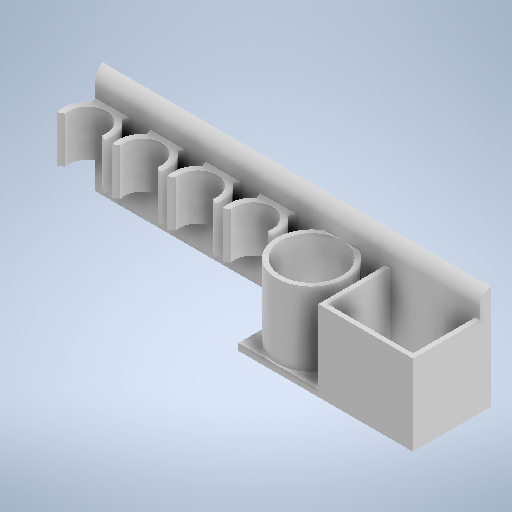
# Autodesk Inventor part: Block-1
Saved by Autodesk Inventor 2025 (Build 290162000, 162)
## iProperties
Created: 2024-07-25
Part Number: Block-1
Material: Generic
Document SubType Name: Modeling
Designer: ethan
Density: 1 g/cm^3
Appearance: Default
Author: ethan
Autodesk Inventor part; units mm, degrees
ref_plane "YZ Plane" through (0, 0, 0) normal (1, 0, 0) x (0, 1, 0)
ref_plane "XZ Plane" through (0, 0, 0) normal (0, 1, 0) x (-1, 0, 0)
ref_plane "XY Plane" through (0, 0, 0) normal (0, 0, 1) x (1, 0, 0)
sketch "Sketch1" plane through (0, 0, 0) normal (0, 1, 0) x (-1, 0, 0)
  arc A0 (-1.6722, -8.0788) -> (-1.6722, 8.0788) centre (0, 0) ccw
  arc A1 (-2.9725, -10.3309) -> (-2.9725, 10.3309) centre (0, 0) ccw
  line L0 (-1.6722, 8.0788) -> (-2.9725, 10.3309)
  line L1 (-1.6722, 8.0788) -> (0.9283, 8.0788) construction
  line L2 (-1.6722, -8.0788) -> (-2.9725, -10.3309)
  line L3 (0, 0) -> (0, -2.9706)
  arc A2 (-1.6722, -32.0788) -> (-1.6722, -15.9212) centre (0, -24) ccw
  arc A3 (-2.9725, -34.3309) -> (-2.9725, -13.6691) centre (0, -24) ccw
  line L4 (-1.6722, -15.9212) -> (-2.9725, -13.6691)
  line L5 (-1.6722, -15.9212) -> (0.9283, -15.9212) construction
  line L6 (-1.6722, -32.0788) -> (-2.9725, -34.3309)
  line L7 (0, -24) -> (0, -26.9706)
  arc A4 (-1.6722, -56.0788) -> (-1.6722, -39.9212) centre (0, -48) ccw
  arc A5 (-2.9725, -58.3309) -> (-2.9725, -37.6691) centre (0, -48) ccw
  line L8 (-1.6722, -39.9212) -> (-2.9725, -37.6691)
  line L9 (-1.6722, -39.9212) -> (0.9283, -39.9212) construction
  line L10 (-1.6722, -56.0788) -> (-2.9725, -58.3309)
  line L11 (0, -48) -> (0, -50.9706)
  arc A6 (-1.6722, -80.0788) -> (-1.6722, -63.9212) centre (0, -72) ccw
  arc A7 (-2.9725, -82.3309) -> (-2.9725, -61.6691) centre (0, -72) ccw
  line L12 (-1.6722, -63.9212) -> (-2.9725, -61.6691)
  line L13 (-1.6722, -63.9212) -> (0.9283, -63.9212) construction
  line L14 (-1.6722, -80.0788) -> (-2.9725, -82.3309)
  line L15 (0, -72) -> (0, -74.9706)
  line L16 (10.75, -99.7274) -> (-2.45, -99.7274) construction
  circle A8 centre (-2.45, -99.7274) radius 13.2 construction
  arc A9 (10.75, -92.1908) -> (10.75, -107.264) centre (-2.45, -99.7274) ccw construction
  circle A10 centre (-2.45, -99.7274) radius 13.2
  arc A11 (10.75, -92.1908) -> (10.75, -107.264) centre (-2.45, -99.7274) ccw
  line L17 (10.75, -120.472) -> (-16.25, -120.472)
  line L18 (-16.25, -120.472) -> (-16.25, -157.572)
  line L19 (-16.25, -157.572) -> (10.75, -157.572)
  line L20 (10.75, -157.572) -> (10.75, -120.472)
  line L21 (-18.25, -159.572) -> (-18.25, -118.472)
  line L22 (-18.25, -118.472) -> (10.75, -118.472)
  line L23 (12.75, -159.572) -> (-18.25, -159.572)
  line L24 (10.75, 0) -> (15.75, 0) construction
  line L25 (8.4709, 6.6186) -> (15.75, 9.268) construction
  line L26 (15.75, 9.268) -> (15.75, -159.572) construction
  line L27 (15.75, -159.572) -> (12.75, -159.572) construction
  line L28 (10.75, -118.472) -> (10.75, -107.264) construction
  line L29 (10.75, -118.472) -> (10.75, -107.264)
  line L30 (10.75, -92.1908) -> (10.75, -79.8019)
  line L31 (8.4709, 6.6186) -> (15.75, 9.268)
  line L32 (15.75, 9.268) -> (15.75, -159.572)
  line L33 (15.75, -159.572) -> (12.75, -159.572)
  line L34 (10.75, -107.264) -> (10.75, -118.472) construction
  line L35 (10.75, -120.472) -> (10.75, -154.7804) construction
  line L36 (8.4709, -6.6186) -> (10.75, -7.4481)
  line L37 (8.4709, -6.6186) -> (10.8963, -6.6186) construction
  line L38 (8.4709, -17.3814) -> (10.75, -16.5519)
  line L39 (8.4709, -30.6186) -> (10.75, -31.4481)
  line L40 (8.4709, -41.3814) -> (10.75, -40.5519)
  line L41 (8.4709, -54.6186) -> (10.75, -55.4481)
  line L42 (8.25, -65.108) -> (10.75, -64.1981)
  line L43 (8.25, -78.892) -> (10.75, -79.8019)
  line L44 (10.75, -16.5519) -> (10.75, -7.4481)
  line L45 (10.75, -7.4481) -> (10.75, -16.5519) construction
  line L46 (10.75, -64.1981) -> (10.75, -55.4481)
  line L47 (10.75, -40.5519) -> (10.75, -31.4481)
  line L48 (10.75, -31.4481) -> (10.75, -40.5519) construction
  line L49 (10.75, -55.4481) -> (10.75, -64.1981) construction
  line L50 (10.75, -79.8019) -> (10.75, -92.1908) construction
  dimension "d1" = 2.5
  dimension "d5" = 24
  dimension "d19" = 20
  constraints: 102 end point, 29 point on circle, 28 collinear, 12 tangent, 11 centre point, 10 parallel, 9 perpendicular, 9 vertical, 7 coincident, 4 horizontal, 2 equal length, 1 concentric, 1 horizontal alignment, 47 other
  measures "d1" radial gap between concentric circles of A0 A1
  measures "d5" distance of point (0, 0) point (0, -24)
  measures "d19" angle of L36 L37
extrude "Extrusion1" add sketch "Sketch1" along normal blind 20
sketch "Sketch2" plane through (0, 20, 0) normal (0, 1, 0) x (1, 0, 0)
  arc A0 (-10.75, 92.1908) -> (-10.75, 107.264) centre (2.45, 99.7274) ccw construction
  line L0 (-10.75, 107.264) -> (-10.75, 118.472) construction
  line L1 (-10.75, 118.472) -> (18.25, 118.472) construction
  line L2 (18.25, 118.472) -> (18.25, 159.572) construction
  line L3 (18.25, 159.572) -> (-15.75, 159.572) construction
  line L4 (-15.75, 159.572) -> (-15.75, -9.268) construction
  line L5 (-15.75, -9.268) -> (-8.4709, -6.6186) construction
  arc A1 (-8.4709, -6.6186) -> (2.9725, -10.3309) centre (0, 0) ccw construction
  line L6 (2.9725, -10.3309) -> (1.6722, -8.0788) construction
  arc A2 (1.6722, 8.0788) -> (1.6722, -8.0788) centre (0, 0) ccw construction
  line L7 (1.6722, 8.0788) -> (2.9725, 10.3309) construction
  arc A3 (2.9725, 10.3309) -> (-8.4709, 6.6186) centre (0, 0) ccw construction
  line L8 (-8.4709, 6.6186) -> (-10.75, 7.4481) construction
  line L9 (-10.75, 7.4481) -> (-10.75, 16.5519) construction
  line L10 (-10.75, 16.5519) -> (-8.4709, 17.3814) construction
  arc A4 (-8.4709, 17.3814) -> (2.9725, 13.6691) centre (0, 24) ccw construction
  line L11 (2.9725, 13.6691) -> (1.6722, 15.9212) construction
  arc A5 (1.6722, 32.0788) -> (1.6722, 15.9212) centre (0, 24) ccw construction
  line L12 (1.6722, 32.0788) -> (2.9725, 34.3309) construction
  arc A6 (2.9725, 34.3309) -> (-8.4709, 30.6186) centre (0, 24) ccw construction
  line L13 (-8.4709, 30.6186) -> (-10.75, 31.4481) construction
  line L14 (-10.75, 31.4481) -> (-10.75, 40.5519) construction
  line L15 (-10.75, 40.5519) -> (-8.4709, 41.3814) construction
  arc A7 (-8.4709, 41.3814) -> (2.9725, 37.6691) centre (0, 48) ccw construction
  line L16 (2.9725, 37.6691) -> (1.6722, 39.9212) construction
  arc A8 (1.6722, 56.0788) -> (1.6722, 39.9212) centre (0, 48) ccw construction
  line L17 (1.6722, 56.0788) -> (2.9725, 58.3309) construction
  arc A9 (2.9725, 58.3309) -> (-8.4709, 54.6186) centre (0, 48) ccw construction
  line L18 (-8.4709, 54.6186) -> (-10.75, 55.4481) construction
  line L19 (-10.75, 55.4481) -> (-10.75, 64.1981) construction
  line L20 (-10.75, 64.1981) -> (-8.25, 65.108) construction
  arc A10 (-8.25, 65.108) -> (2.9725, 61.6691) centre (0, 72) ccw construction
  line L21 (2.9725, 61.6691) -> (1.6722, 63.9212) construction
  arc A11 (1.6722, 80.0788) -> (1.6722, 63.9212) centre (0, 72) ccw construction
  line L22 (1.6722, 80.0788) -> (2.9725, 82.3309) construction
  arc A12 (2.9725, 82.3309) -> (-8.25, 78.892) centre (0, 72) ccw construction
  line L23 (-8.25, 78.892) -> (-10.75, 79.8019) construction
  line L24 (-10.75, 79.8019) -> (-10.75, 92.1908) construction
  line L25 (-10.75, 120.472) -> (-10.75, 157.572) construction
  line L26 (-10.75, 157.572) -> (16.25, 157.572) construction
  line L27 (16.25, 157.572) -> (16.25, 120.472) construction
  line L28 (16.25, 120.472) -> (-10.75, 120.472) construction
  circle A13 centre (2.45, 99.7274) radius 13.2 construction
  line L29 (-15.75, -9.268) -> (-10.75, -9.268)
  line L30 (-10.75, -9.268) -> (-10.75, 159.572)
  line L31 (-10.75, 159.572) -> (-15.75, 159.572)
  line L32 (-15.75, 159.572) -> (-15.75, -9.268)
  line L33 (-15.75, -9.268) -> (-8.4709, -6.6186) projected
  line L34 (-10.75, -7.4481) -> (-15.75, -9.268)
  constraints: 10 end point, 3 point on line, 2 parallel, 1 collinear, 1 horizontal, 1 perpendicular
extrude "Extrusion2" add sketch "Sketch2" along normal blind 10 contours L32 L31 L30 L33
sketch "Sketch3" plane through (0, 0, 0) normal (0, -1, 0) x (1, 0, 0)
  arc A0 (-10.75, -107.264) -> (-10.75, -92.1908) centre (2.45, -99.7274) ccw projected
  line L0 (-10.75, -79.8019) -> (-10.75, -92.1908) projected
  line L1 (-8.25, -78.892) -> (-10.75, -79.8019) projected
  arc A1 (-8.25, -78.892) -> (2.9725, -82.3309) centre (0, -72) ccw projected
  line L2 (1.6722, -80.0788) -> (2.9725, -82.3309) projected
  arc A2 (1.6722, -63.9212) -> (1.6722, -80.0788) centre (0, -72) ccw projected
  line L3 (2.9725, -61.6691) -> (1.6722, -63.9212) projected
  arc A3 (2.9725, -61.6691) -> (-8.25, -65.108) centre (0, -72) ccw projected
  line L4 (-10.75, -64.1981) -> (-8.25, -65.108) projected
  line L5 (-10.75, -55.4481) -> (-10.75, -64.1981) projected
  line L6 (-8.4709, -54.6186) -> (-10.75, -55.4481) projected
  arc A4 (-8.4709, -54.6186) -> (2.9725, -58.3309) centre (0, -48) ccw projected
  line L7 (1.6722, -56.0788) -> (2.9725, -58.3309) projected
  arc A5 (1.6722, -39.9212) -> (1.6722, -56.0788) centre (0, -48) ccw projected
  line L8 (2.9725, -37.6691) -> (1.6722, -39.9212) projected
  arc A6 (2.9725, -37.6691) -> (-8.4709, -41.3814) centre (0, -48) ccw projected
  line L9 (-10.75, -40.5519) -> (-8.4709, -41.3814) projected
  line L10 (-10.75, -31.4481) -> (-10.75, -40.5519) projected
  line L11 (-8.4709, -30.6186) -> (-10.75, -31.4481) projected
  arc A7 (-8.4709, -30.6186) -> (2.9725, -34.3309) centre (0, -24) ccw projected
  line L12 (1.6722, -32.0788) -> (2.9725, -34.3309) projected
  arc A8 (1.6722, -15.9212) -> (1.6722, -32.0788) centre (0, -24) ccw projected
  line L13 (2.9725, -13.6691) -> (1.6722, -15.9212) projected
  arc A9 (2.9725, -13.6691) -> (-8.4709, -17.3814) centre (0, -24) ccw projected
  line L14 (-10.75, -16.5519) -> (-8.4709, -17.3814) projected
  line L15 (-10.75, -7.4481) -> (-10.75, -16.5519) projected
  line L16 (-8.4709, -6.6186) -> (-10.75, -7.4481) projected
  arc A10 (-8.4709, -6.6186) -> (2.9725, -10.3309) centre (0, 0) ccw projected
  line L17 (1.6722, -8.0788) -> (2.9725, -10.3309) projected
  arc A11 (1.6722, 8.0788) -> (1.6722, -8.0788) centre (0, 0) ccw projected
  line L18 (2.9725, 10.3309) -> (1.6722, 8.0788) projected
  arc A12 (2.9725, 10.3309) -> (-8.4709, 6.6186) centre (0, 0) ccw projected
  line L19 (-15.75, 9.268) -> (-8.4709, 6.6186) projected
  line L20 (-15.75, -159.572) -> (-15.75, 9.268) projected
  line L21 (18.25, -159.572) -> (-15.75, -159.572) projected
  line L22 (18.25, -118.472) -> (18.25, -159.572) projected
  line L23 (-10.75, -118.472) -> (18.25, -118.472) projected
  line L24 (-10.75, -107.264) -> (-10.75, -118.472) projected
  line L25 (-10.75, -120.472) -> (-10.75, -157.572) projected
  line L26 (16.25, -120.472) -> (-10.75, -120.472) projected
  line L27 (16.25, -157.572) -> (16.25, -120.472) projected
  line L28 (-10.75, -157.572) -> (16.25, -157.572) projected
  circle A13 centre (2.45, -99.7274) radius 13.2 projected
  line L29 (2.45, -84.5274) -> (-15.75, -84.5274)
  arc A14 (-10.75, -107.264) -> (-10.75, -92.1908) centre (2.45, -99.7274) ccw projected
  line L30 (-15.75, -84.5274) -> (-10.75, -84.5274)
  line L31 (-10.75, -84.5274) -> (-10.75, -159.572)
  line L32 (-10.75, -159.572) -> (-15.75, -159.572)
  line L33 (-15.75, -159.572) -> (-15.75, -84.5274)
  line L34 (-15.75, -84.5274) -> (-10.75, -84.5274)
  line L35 (-10.75, -84.5274) -> (-10.75, -7.4481)
  line L36 (-10.75, -7.4481) -> (-15.75, -7.4481)
  line L37 (-15.75, -7.4481) -> (-15.75, -84.5274)
  line L38 (-15.75, -159.572) -> (-15.75, 9.268) projected
  line L39 (-10.75, -7.4481) -> (-15.75, -7.4481)
  line L40 (-15.75, -7.4481) -> (-15.75, 9.268)
  line L41 (-15.75, 9.268) -> (-10.75, 9.268)
  line L42 (-10.75, 9.268) -> (-10.75, -7.4481)
  point P0 (-10.75, 7.4481)
  constraints: 26 end point, 6 parallel, 4 perpendicular, 3 horizontal, 2 point on line, 1 point on circle, 1 tangent
extrude "Extrusion3" add sketch "Sketch3" along normal blind 15 contours L31 A0 | L24 L31 L25 L21 L20 L29 L0 | L23 L22 L21 L31 L28 L27 L26 | L29 L20 L36 L15 L35 L10 L5 L0 | L20 L19 L42 L36
sketch "Sketch4" plane through (0, -15, 0) normal (0, -1, 0) x (1, 0, 0)
  line L0 (-10.75, 7.4481) -> (-15.75, 9.268) construction
  line L1 (-15.75, 9.268) -> (-15.75, -159.572) construction
  line L2 (-15.75, -159.572) -> (18.25, -159.572) construction
  line L3 (18.25, -159.572) -> (18.25, -118.472) construction
  line L4 (18.25, -118.472) -> (-10.75, -118.472) construction
  line L5 (-10.75, -118.472) -> (-10.75, -107.264) construction
  arc A0 (-10.75, -107.264) -> (-10.75, -92.1908) centre (2.45, -99.7274) ccw construction
  line L6 (-10.75, -92.1908) -> (-10.75, 7.4481) construction
  circle A1 centre (2.45, -99.7274) radius 13.2 construction
  line L7 (-10.75, -157.572) -> (-10.75, -120.472) construction
  line L8 (-10.75, -120.472) -> (16.25, -120.472) construction
  line L9 (16.25, -120.472) -> (16.25, -157.572) construction
  line L10 (16.25, -157.572) -> (-10.75, -157.572) construction
  line L11 (-10.75, 7.4481) -> (-10.75, -7.4481) construction
  line L12 (-8.4709, -6.6186) -> (-10.75, -7.4481) construction
  arc A2 (-8.4709, -6.6186) -> (2.9725, -10.3309) centre (0, 0) ccw construction
  line L13 (1.6722, -8.0788) -> (2.9725, -10.3309) construction
  arc A3 (1.6722, 8.0788) -> (1.6722, -8.0788) centre (0, 0) ccw construction
  line L14 (2.9725, 10.3309) -> (1.6722, 8.0788) construction
  arc A4 (2.9725, 10.3309) -> (-8.4709, 6.6186) centre (0, 0) ccw construction
  line L15 (-10.75, 7.4481) -> (-8.4709, 6.6186) construction
  line L16 (-10.75, -16.5519) -> (-10.75, -31.4481) construction
  line L17 (-8.4709, -30.6186) -> (-10.75, -31.4481) construction
  arc A5 (-8.4709, -30.6186) -> (2.9725, -34.3309) centre (0, -24) ccw construction
  line L18 (1.6722, -32.0788) -> (2.9725, -34.3309) construction
  arc A6 (1.6722, -15.9212) -> (1.6722, -32.0788) centre (0, -24) ccw construction
  line L19 (2.9725, -13.6691) -> (1.6722, -15.9212) construction
  arc A7 (2.9725, -13.6691) -> (-8.4709, -17.3814) centre (0, -24) ccw construction
  line L20 (-10.75, -16.5519) -> (-8.4709, -17.3814) construction
  line L21 (-10.75, -40.5519) -> (-10.75, -55.4481) construction
  line L22 (-8.4709, -54.6186) -> (-10.75, -55.4481) construction
  arc A8 (-8.4709, -54.6186) -> (2.9725, -58.3309) centre (0, -48) ccw construction
  line L23 (1.6722, -56.0788) -> (2.9725, -58.3309) construction
  arc A9 (1.6722, -39.9212) -> (1.6722, -56.0788) centre (0, -48) ccw construction
  line L24 (2.9725, -37.6691) -> (1.6722, -39.9212) construction
  arc A10 (2.9725, -37.6691) -> (-8.4709, -41.3814) centre (0, -48) ccw construction
  line L25 (-10.75, -40.5519) -> (-8.4709, -41.3814) construction
  arc A11 (1.6722, -63.9212) -> (1.6722, -80.0788) centre (0, -72) ccw construction
  line L26 (-10.75, -64.1981) -> (-10.75, -79.8019) construction
  line L27 (-8.25, -78.892) -> (-10.75, -79.8019) construction
  arc A12 (-8.25, -78.892) -> (2.9725, -82.3309) centre (0, -72) ccw construction
  line L28 (1.6722, -80.0788) -> (2.9725, -82.3309) construction
  arc A13 (1.6722, -63.9212) -> (1.6722, -80.0788) centre (0, -72) ccw construction
  line L29 (2.9725, -61.6691) -> (1.6722, -63.9212) construction
  arc A14 (2.9725, -61.6691) -> (-8.25, -65.108) centre (0, -72) ccw construction
  line L30 (-10.75, -64.1981) -> (-8.25, -65.108) construction
  line L31 (-15.75, 9.268) -> (18.25, 9.268)
  line L32 (18.25, 9.268) -> (18.25, -159.572)
  line L33 (-15.75, -159.572) -> (18.25, -159.572)
  line L34 (-15.75, -159.572) -> (-15.75, 9.268)
  circle A15 centre (0, 0) radius 8.25
  circle A16 centre (0, -24) radius 8.25
  circle A17 centre (0, -48) radius 8.25
  circle A18 centre (0, -72) radius 8.25
  line L35 (-15.75, -83.7856) -> (18.25, -83.7856)
  point P0 (2.45, -84.5274)
  constraints: 10 end point, 4 coincident, 3 point on line, 2 collinear, 2 perpendicular, 1 point on circle, 12 other
extrude "Extrusion4" add sketch "Sketch4" against normal blind 3 contours L35 L32 L33 L34
fillet "Fillet1" radius 5 1 edges at (-10.75, 30, -76.0619)
body "Solid1"
